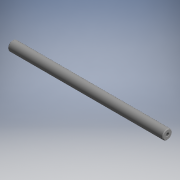
# Autodesk Inventor part: AETTF8-130-M3-N3
Saved by Autodesk Inventor 2017.3 (Build 213256000, 256)
## iProperties
Part Number: AETTF8-130-M3-N3
Material: Generic
Catalog Web Link: www.cadenas.de
Description: NETF, ETKF, PETF, SETF, AETTF, ABETTF-Circular Posts - Both Ends Tapped - Thread Diameter Configurable
Vendor: MISUMI
Document SubType Name: Modeling
Designer: partserver
Manufacturer: MISUMI
Mass: 6.4469 g
Surface Area: 34.7971 cm^2
Volume: 6.4469 cm^3
Density: 1 g/cm^3
Appearance: PSOLRGB-175-175-175
Category: PARTsolutions
Company: MISUMI
Title: AETTF8-130-M3-N3
Author: Cadenas PARTsolutions
Comments: Circular Posts - Both Ends Tapped - Thread Diameter Configurable
PSOL_IDENT_0: {$CADENAS_DATA\23d-libs\misumi\metric\19_posts_stands\petf.prj},251 {VTYP=3D},{NB=AETTF8-130-M3-N3},
PSOL_IDENT_1: {LINA=AETTF8-130-M3-N3},{NN=NETF, ETKF, PETF, SETF, AETTF, ABETTF},{DATE=02.06.2021 23:49:04},{GEOMD
PSOL_IDENT_2: ATE=26.03.2021 07:55:44},{VERSION=},{LINEID=60},{WBVAR=MAT,ST,L,M,N,ALT4,ALT5,ALT1,ALT6,ALT2,HL},{WB
PSOL_IDENT_3: NUMERIC=L,M,N,HL}  {NB=AETTF8-130-M3-N3},{LINA=AETTF8-130-M3-N3},{KT=DUMMY},{PN=AETTF8-130-M3-N3},{T
PSOL_IDENT_4: YPE=AETTF},{MAT=A2017},{MATALG= 'LCS','Low Carbon Steel', 'SUS304', 'SUS304', 'A2017', '2017 Aluminu
PSOL_IDENT_5: m Alloy' },{ST=CA},{STALG= 'CA', 'Clear Anodize' , 'BA', 'Black Anodize' },{D=8},{L=130.0},{M=3.0},{
PSOL_IDENT_6: M1=[3,4,5]},{MPITCH=0.500},{MDEPT=9.00},{MAV=3},{N=3.0},{N1=[3,4,5]},{NPITCH=0.500},{NDEPT=9.00},{NA
PSOL_IDENT_7: V=4},{ALT4=},{ALT4ALG='','w/o MD (Left End Change The Effective Tap Depth)','MD','with MD (Left End
PSOL_IDENT_8: Change The Effective Tap Depth)'},{ALT4PN=-M3},{ALT5=},{ALT5ALG='','w/o ND (Right End Change The Eff
PSOL_IDENT_9: ective Tap Depth)','ND','with ND (Right End Change The Effective Tap Depth)'},{ALT5PN=-N3},{ALT1=},{
PSOL_IDENT_10: LKC=±0.1},{LALG=[15:400/0.5]},{LMIN=15.0},{LMIN1=15},{LMIN2=12},{LMIN21=120},{LMIN22=150},{LMIN23=15
PSOL_IDENT_11: 0},{LMIN3=15},{LMAX=400},{ALT6=},{ALT6ALG= '', 'w/o LVC (L Dimension Accuracy Change)', 'LVC', 'with
PSOL_IDENT_12: LVC (L Dimension Accuracy Change)'},{ALT6PN=},{ALT2=},{ALT2ALG= '', 'w/o HL (Through Hole for Hex W
PSOL_IDENT_13: rench)', '-HL', 'with HL (Through Hole for Hex Wrench)' },{ALT2PN=},{HL=0},{HLALG=0},{HLMIN=7},{HLMA
PSOL_IDENT_14: X=123},{DD=0.0},{DD1=2.5}
NB: AETTF8-130-M3-N3
NN: NETF, ETKF, PETF, SETF, AETTF, ABETTF
NT: Circular Posts - Both Ends Tapped - Thread Diameter Configurable
NBSYN: $PN.
LINA: AETTF8-130-M3-N3
CATALOG: Misumi
PN: AETTF8-130-M3-N3
TYPE: AETTF
MAT: 2017 Aluminum Alloy
ST: Clear Anodize
D: 8
L: 130
M: 3
N: 3
ALT4: w/o MD (Left End Change The Effective Tap Depth)
ALT5: w/o ND (Right End Change The Effective Tap Depth)
ALT1: w/o LKC (L Dimension Tolerance Change)
LKC: ±0.1
ALT6: w/o LVC (L Dimension Accuracy Change)
ALT2: w/o HL (Through Hole for Hex Wrench)
HL: 0
DD: 0
SUPPLIER: MISUMI
ARTICLENO: AETTF8-130-M3-N3
BOMINFO: AETTF8-130-M3-N3
CREATOR: CADENAS GmbH
Autodesk Inventor part; units mm, degrees
ref_plane "YZ Plane" through (0, 0, 0) normal (1, 0, 0) x (0, 1, 0)
ref_plane "XZ Plane" through (0, 0, 0) normal (0, 1, 0) x (-1, 0, 0)
ref_plane "XY Plane" through (0, 0, 0) normal (0, 0, 1) x (1, 0, 0)
sketch "Sketch_1" plane through (0, 0, 0) normal (0, 0, 1) x (1, 0, 0)
  line L0 (130, 0) -> (0, 0)
  line L1 (0, 0) -> (0, 3.5)
  line L2 (0, 3.5) -> (0.5, 4)
  line L3 (0.5, 4) -> (129.5, 4)
  line L4 (129.5, 4) -> (130, 3.5)
  line L5 (130, 3.5) -> (130, 0)
  line L6 (130, 0) -> (0, 0)
  constraints: 14 end point
revolve "Revolution1" add sketch "Sketch_1" angle 360 about axis through (130, 0, 0) along (1, 0, 0)
sketch "Sketch2" plane through (0, 0, 0) normal (-1, 0, 0) x (0, 0, 1)
  point P0 (0, 0)
hole "Hole1" at (0, 0, 0) direction (1, 0, 0) diameter 2.459 depth 8.2901 tip angle 120 countersink diameter 3 countersink angle 90 thread size "M3x0.5" class "6H" standard "ISO Metric profile"
sketch "Sketch3" plane through (130, 0, 0) normal (1, 0, 0) x (0, 0, -1)
  point P0 (0, 0)
hole "Hole2" at (130, 0, 0) direction (-1, 0, 0) diameter 2.459 depth 8.2901 tip angle 120 countersink diameter 3 countersink angle 90 thread size "M3x0.5" class "6H" standard "ISO Metric profile"
body "Solid1"
